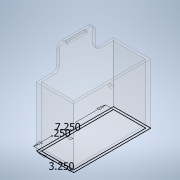
# Autodesk Inventor part: Part3
Saved by Autodesk Inventor 2022 (Build 260153000, 153)
## iProperties
Created: 2022-12-07
Part Number: Part3
Material: Polycarbonate, Clear
Document SubType Name: Modeling
Designer: S135320
Mass: 764.764 g
Surface Area: 2044.35 cm^2
Volume: 637.303 cm^3
Density: 1.2 g/cm^3
Appearance: Polycarbonate - Clear
Author: S135320
Autodesk Inventor part; units mm, degrees
ref_plane "YZ Plane" through (0, 0, 0) normal (1, 0, 0) x (0, 1, 0)
ref_plane "XZ Plane" through (0, 0, 0) normal (0, 1, 0) x (-1, 0, 0)
ref_plane "XY Plane" through (0, 0, 0) normal (0, 0, 1) x (1, 0, 0)
sketch "Sketch1" plane through (0, 0, 0) normal (0, 1, 0) x (-1, 0, 0)
  line L0 (0, 0) -> (82.55, 0)
  line L1 (82.55, 0) -> (82.55, -184.15)
  line L2 (82.55, -184.15) -> (0, -184.15)
  line L3 (0, -184.15) -> (0, 0)
  line L4 (88.9, -190.5) -> (88.9, 6.35)
  line L5 (88.9, 6.35) -> (-6.35, 6.35)
  line L6 (-6.35, 6.35) -> (-6.35, -190.5)
  line L7 (-6.35, -190.5) -> (88.9, -190.5)
  dimension "d0" = 184.15
  dimension "d1" = 82.55
  dimension "d2" = 6.35
  constraints: 16 end point, 4 parallel, 2 perpendicular, 1 horizontal, 3 other
  measures "d0" distance of L0.end L1.end
  measures "d1" distance of L0.start L0.end
  measures "d2" distance between parallel lines of L4 L1
extrude "Extrusion1" add sketch "Sketch1" along normal blind 6.35 contours L0 L1 L2 L3
extrude "Extrusion2" add sketch "Sketch1" along normal blind 152.4
sketch "Sketch2" plane through (-88.9, 0, -190.5) normal (-1, 0, 0) x (0, 0, 1)
  line L0 (52.5316, 92.2462) -> (144.3184, 92.2462)
  line L1 (144.3184, 92.2462) -> (144.3184, 212.5538)
  line L2 (144.3184, 212.5538) -> (52.5316, 212.5538)
  line L3 (52.5316, 212.5538) -> (52.5316, 92.2462)
  line L4 (190.5, 152.4) -> (6.35, 152.4) projected
  line L5 (52.5316, 92.2462) -> (144.3184, 212.5538) construction
  line L6 (144.3184, 92.2462) -> (52.5316, 212.5538) construction
  point P0 (190.5, 0)
  point P1 (98.425, 152.4)
  point P2 (52.5316, 152.4)
  point P3 (144.3184, 152.4)
  constraints: 12 end point, 3 midpoint, 2 parallel, 1 horizontal, 1 perpendicular
extrude "Extrusion3" add sketch "Sketch2" against normal blind 6.35 contours L3 L2 L1 L4
fillet "Fillet1" radius 12.7 4 edges at (-85.725, 212.5538, -46.1816) (-85.725, 152.4, -46.1816) (-85.725, 212.5538, -137.9684) (-85.725, 152.4, -137.9684)
sketch "Sketch3" plane through (-82.55, 6.35, 0) normal (1, 0, 0) x (0, 0, -1)
  line L0 (125.2684, 206.2038) -> (58.8816, 206.2038) projected
  line L1 (92.075, 206.2038) -> (92.075, 193.6256)
  line L2 (67.0657, 201.1795) -> (117.0843, 201.1795)
  line L3 (117.0843, 201.1795) -> (117.0843, 196.1885)
  line L4 (117.0843, 196.1885) -> (67.0657, 196.1885)
  line L5 (67.0657, 196.1885) -> (67.0657, 201.1795)
  line L6 (67.0657, 201.1795) -> (117.0843, 196.1885) construction
  line L7 (117.0843, 201.1795) -> (67.0657, 196.1885) construction
  point P0 (0, -6.35)
  point P1 (92.075, 198.684)
  constraints: 14 end point, 3 midpoint, 2 parallel, 1 horizontal, 1 perpendicular, 1 point on line, 1 vertical
extrude "Extrusion4" cut sketch "Sketch3" against normal blind 6.35
sketch "Sketch4" plane through (6.35, 0, 6.35) normal (1, 0, 0) x (0, 0, -1)
  line L0 (0, 152.4) -> (196.85, 152.4) projected
  line L1 (98.425, 152.4) -> (98.425, 129.719)
  circle A0 centre (98.425, 141.0595) radius 4.0936
  point P0 (6.35, 0)
  constraints: 2 end point, 2 midpoint, 1 centre point, 1 vertical
extrude "Extrusion5" cut sketch "Sketch4" against normal up to surface (6.35 mm away)
body "Solid1"
